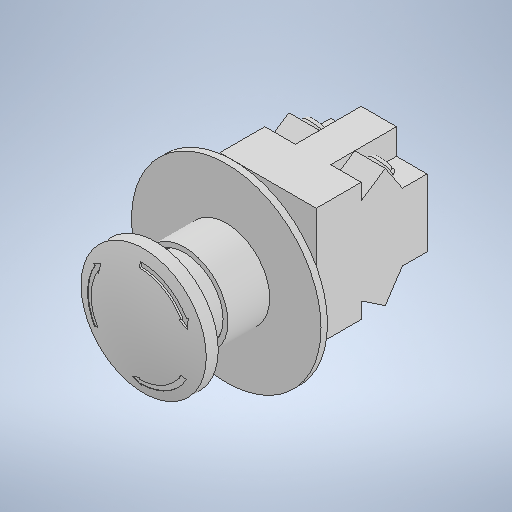
# Autodesk Inventor part: EmergencyStop
Saved by Autodesk Inventor 2025.1 (Build 291241020, 241B)
## iProperties
Created: 2024-09-11
Part Number: EmergencyStop
Material: 一般
Document SubType Name: Modeling
Designer: 8326d
Density: 1 g/cm^3
Appearance: 既定
Author: 8326d
Autodesk Inventor part; units mm, degrees
ref_plane "YZ Plane" through (0, 0, 0) normal (1, 0, 0) x (0, 1, 0)
ref_plane "XZ Plane" through (0, 0, 0) normal (0, 1, 0) x (-1, 0, 0)
ref_plane "XY Plane" through (0, 0, 0) normal (0, 0, 1) x (1, 0, 0)
sketch "スケッチ1" plane through (0, 0, 0) normal (0, 0, 1) x (1, 0, 0)
  line L0 (-15, -18.5) -> (15, -18.5)
  line L1 (15, -18.5) -> (15, 18.5)
  line L2 (15, 18.5) -> (-15, 18.5)
  line L3 (-15, 18.5) -> (-15, -18.5)
  line L4 (-15, -18.5) -> (15, 18.5) construction
  line L5 (15, -18.5) -> (-15, 18.5) construction
  point P0 (0, 0)
  dimension "d0" = 30
  dimension "d1" = 37
  constraints: 12 end point, 2 midpoint, 2 parallel, 1 horizontal, 1 perpendicular
  measures "d0" distance of L2.end L1.end
  measures "d1" distance of L1.end L0.end
extrude "押し出し1" add sketch "スケッチ1" along normal blind 34.5
sketch "スケッチ2" plane through (15, -18.5, 0) normal (1, 0, 0) x (0, 0, -1)
  line L0 (0, 0) -> (0, 37) projected
  line L1 (0, 37) -> (-34.5, 37) projected
  line L2 (-34.5, 0) -> (-34.5, 37) projected
  line L3 (0, 0) -> (-34.5, 0) projected
  line L4 (-20.5, 37) -> (-20.5, 0)
  line L5 (-20.5, 32) -> (-13, 37)
  line L6 (-13, 37) -> (-7.6667, 29)
  line L7 (-7.6667, 29) -> (0, 29)
  point P0 (0, 18.5)
  dimension "d4" = 14
  dimension "d5" = 8
  dimension "d6" = 7.5
  dimension "d7" = 5
  constraints: 8 end point, 5 point on line, 2 perpendicular, 1 horizontal
  measures "d4" distance between parallel lines of L2 L4
  measures "d5" distance between parallel lines of L1 L7
  measures "d6" distance from line of L4 L5.end
  measures "d7" distance from line of L1 L5.start
extrude "押し出し2" cut sketch "スケッチ2" against normal blind 9.5 contours L7 L6 L1 L0 | L4 L1 L5
sketch "スケッチ3" plane through (15, 10.5, 7.6667) normal (0, 0.5547002, -0.8320503) x (-1, 0, 0)
  line L0 (0, 0) -> (0, 9.6148) projected
  line L1 (0, 0) -> (9.5, 0) projected
  line L2 (9.5, 0) -> (9.5, 9.6148) projected
  line L3 (9.5, 9.6148) -> (0, 9.6148) projected
  circle A0 centre (4.75, 4.8074) radius 3.5
  point P0 (15, -12.9892)
  point P1 (9.5, 4.8074)
  point P2 (4.75, 9.6148)
  dimension "d10" = 7
  constraints: 2 midpoint, 1 centre point, 1 horizontal alignment, 1 vertical alignment
  measures "d10" diameter of A0
extrude "押し出し3" add sketch "スケッチ3" along normal blind 2 contours A0
fillet "フィレット1" radius 1 1 edges at (13.75, 15.6094, 8.6692)
sketch "スケッチ4" plane through (10.25, 15.6094, 8.6692) normal (0, 0.5547002, -0.8320503) x (-1, 0, 0)
  circle A0 centre (0, 0) radius 3.5 projected
  circle A1 centre (0, 0) radius 2.5 projected
  line L0 (-3.5, 0.75) -> (3.5, 0.75)
  line L1 (3.5, 0.75) -> (3.5, -0.75)
  line L2 (3.5, -0.75) -> (-3.5, -0.75)
  line L3 (-3.5, -0.75) -> (-3.5, 0.75)
  line L4 (-3.5, 0.75) -> (3.5, -0.75) construction
  line L5 (3.5, 0.75) -> (-3.5, -0.75) construction
  line L6 (0.75, 2.5) -> (-0.75, 2.5)
  line L7 (-0.75, 2.5) -> (-0.75, -2.5)
  line L8 (-0.75, -2.5) -> (0.75, -2.5)
  line L9 (0.75, -2.5) -> (0.75, 2.5)
  circle A2 centre (0, 0) radius 3.5 projected
  line L10 (0.75, 2.5) -> (-0.75, -2.5) construction
  line L11 (-0.75, 2.5) -> (0.75, -2.5) construction
  point P0 (10.25, -17.7966)
  point P1 (3.5, 0)
  point P2 (0, 2.5)
  point P3 (0.75, -0.75)
  point P4 (0.75, 0.75)
  point P5 (-0.75, 0.75)
  point P6 (-0.75, -0.75)
  dimension "d14" = 1.5
  dimension "d15" = 1.5
  constraints: 24 end point, 6 midpoint, 4 parallel, 2 horizontal, 2 perpendicular, 1 horizontal alignment, 1 vertical alignment, 2 other
  measures "d14" distance between parallel lines of L2 L0
  measures "d15" distance between parallel lines of L7 L9
extrude "押し出し4" cut sketch "スケッチ4" against normal blind 1.2 contours A0 L2 A1 L0 | L1 L2 A0 | A0 L0 L1 | L0 A1 L2 A0 | A0 L3 L0 | A1 L2 L9 L0 | L2 L3 A0 | L0 L7 L2 A1 | L9 L0 L7 A1 | A1 L6 L9 | L9 L2 L7 L0 | L9 L8 A1 | A1 L7 L2 L9 | L7 L6 A1 | A1 L8 L7
mirror "ミラー1" about plane through (0, 0, 0) normal (0, 1, 0) of "押し出し3", "押し出し4", "フィレット1", "押し出し2"
mirror "ミラー2" about plane through (0, 0, 0) normal (1, 0, 0) of "押し出し3", "押し出し4", "フィレット1", "押し出し2", "ミラー1"
sketch "スケッチ5" plane through (0, 0, 34.5) normal (0, 0, 1) x (1, 0, 0)
  circle A0 centre (0, 0) radius 12
  dimension "d18" = 24
  constraints: 1 centre point, 1 coincident
  measures "d18" diameter of A0
extrude "押し出し5" add sketch "スケッチ5" along normal blind 8
sketch "スケッチ6" plane through (0, 0, 42.5) normal (0, 0, 1) x (1, 0, 0)
  circle A0 centre (0, 0) radius 10.75
  dimension "d21" = 21.5
  constraints: 1 centre point, 1 coincident
  measures "d21" diameter of A0
extrude "押し出し6" add sketch "スケッチ6" along normal blind 10
sketch "スケッチ7" plane through (0, 0, 52.5) normal (0, 0, 1) x (1, 0, 0)
  circle A0 centre (0, 0) radius 8
  dimension "d24" = 16
  constraints: 1 centre point, 1 coincident
  measures "d24" diameter of A0
extrude "押し出し7" add sketch "スケッチ7" along normal blind 7
sketch "スケッチ8" plane through (0, 0, 59.5) normal (0, 0, 1) x (1, 0, 0)
  circle A0 centre (0, 0) radius 11.5
  dimension "d27" = 23
  constraints: 1 centre point, 1 coincident
  measures "d27" diameter of A0
extrude "押し出し8" add sketch "スケッチ8" along normal blind 12
sketch "スケッチ9" plane through (0, 0, 0) normal (0, 1, 0) x (-1, 0, 0)
  line L0 (11.5, 71.5) -> (-11.5, 71.5) projected
  line L1 (-19.5, 71.5) -> (19.5, 71.5)
  line L2 (-19.5, 71.5) -> (19.5, 71.5) construction
  line L3 (-19.5, 71.5) -> (-17.5, 71.5)
  line L4 (-17.5, 71.5) -> (-17.5, 69.5)
  line L5 (-17.5, 69.5) -> (-19.5, 69.5)
  line L6 (-19.5, 69.5) -> (-19.5, 71.5)
  arc A0 (19.5, 73.2428) -> (-19.5, 73.2428) centre (0, 16.5) ccw
  line L7 (-19.5, 73.2428) -> (-19.5, 71.5)
  line L8 (0, 71.5) -> (0, 76.5)
  point P0 (0, 0)
  dimension "d30" = 39
  dimension "d31" = 0
  dimension "d32" = 2
  dimension "d33" = 2
  dimension "d34" = 5
  dimension "d35" = 60
  constraints: 16 end point, 3 horizontal, 3 midpoint, 3 parallel, 3 point on circle, 3 vertical alignment, 1 centre point, 1 collinear, 1 perpendicular, 1 vertical
  measures "d30" distance of L1.start L1.end
  measures "d31" distance between parallel lines of L1 L2
  measures "d32" distance of L4.end L5.end
  measures "d33" distance of L3.end L4.end
  measures "d34" distance from line of L0 L8.end
  measures "d35" radius of A0
revolve "回転1" add sketch "スケッチ9" angle 360 about axis through (0, 0, 71.5) along (0, 0, 1)
sketch "スケッチ10" plane through (0, 0, 42.5) normal (0, 0, 1) x (1, 0, 0)
  circle A0 centre (0, 0) radius 14
  dimension "d37" = 28
  constraints: 1 centre point, 1 coincident
  measures "d37" diameter of A0
extrude "押し出し9" add sketch "スケッチ10" along normal blind 3 and the other way blind 4
sketch "スケッチ11" plane through (0, 0, 45.5) normal (0, 0, 1) x (1, 0, 0)
  circle A0 centre (0, 0) radius 29.5
  dimension "d42" = 59
  constraints: 1 centre point, 1 coincident
  measures "d42" diameter of A0
extrude "押し出し10" add sketch "スケッチ11" along normal blind 2
sketch "スケッチ12" plane through (0, 0, 47.5) normal (0, 0, 1) x (1, 0, 0)
  circle A0 centre (0, 0) radius 14 projected
  circle A1 centre (0, 0) radius 14 projected
  circle A2 centre (0, 0) radius 12 projected
  circle A3 centre (0, 0) radius 13.5
  dimension "d45" = 27
  constraints: 1 centre point, 1 coincident
  measures "d45" diameter of A3
extrude "押し出し11" add sketch "スケッチ12" along normal blind 13 contours A3
ref_plane "作業平面1" through (0, 0, 76.5) normal (0, 0, -1) x (-1, 0, 0)
sketch "スケッチ13" plane through (0, 0, 76.5) normal (0, 0, -1) x (-1, 0, 0)
  arc A0 (12.9904, -7.5) -> (12.9904, 7.5) centre (0, 0) ccw
  line L0 (0, 0) -> (12.9904, 7.5) construction
  line L1 (0, 0) -> (12.9904, -7.5) construction
  arc A1 (14.2894, -8.25) -> (14.2894, 8.25) centre (0, 0) ccw
  line L2 (12.9904, -7.5) -> (14.2894, -8.25)
  line L3 (14.2894, 8.25) -> (12.9904, 7.5)
  line L4 (14.7224, 8.5) -> (12.5574, 7.25)
  line L5 (12.5574, 7.25) -> (12.217, 9.9402)
  line L6 (12.217, 9.9402) -> (14.7224, 8.5)
  point P0 (15, 0)
  point P1 (13.6399, 7.875)
  point P2 (12.9904, 7.5)
  point P3 (14.2894, 8.25)
  dimension "d49" = 60
  dimension "d50" = 15
  dimension "d51" = 1.5
  dimension "d52" = 15.75
  dimension "d53" = 2.5
  dimension "d54" = 2.5
  constraints: 14 end point, 5 point on circle, 2 centre point, 2 collinear, 2 midpoint, 1 coincident, 1 horizontal alignment, 1 point on line
  measures "d49" angle of L1 L0
  measures "d50" radius of A0
  measures "d51" radial gap between concentric circles of A0 A1
  measures "d52" distance of point (0, 0) L5.end
  measures "d53" distance of L4.start L4.end
  measures "d54" distance from line of L3 L5.end
extrude "押し出し12" cut sketch "スケッチ13" along normal blind 2.5
pattern_circular "円形状パターン1" count 3 over 360 about axis through (0, 0, -10) along (0, 0, 1) of "押し出し12"
equation "\"d15\" = d14"
